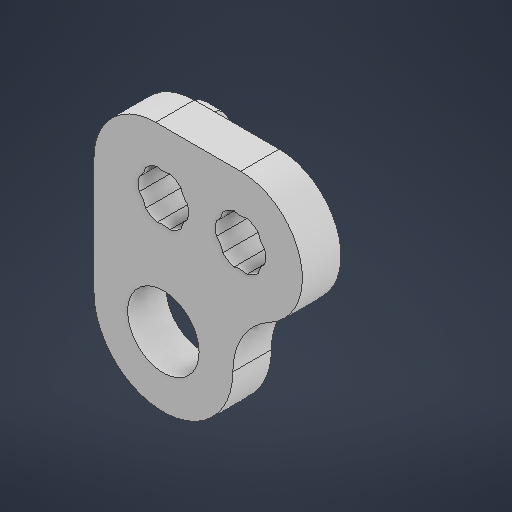
# Autodesk Inventor part: left_holder
Saved by Autodesk Inventor 2026.1 (Build 301233020, 233B)
## iProperties
Created: 2025-12-21
Part Number: left_holder
Material: Ogólny
Document SubType Name: Modeling
Designer: maciej
Density: 1 g/cm^3
Appearance: Domyślna
Author: maciej
Autodesk Inventor part; units mm, degrees
ref_plane "YZ Plane" through (0, 0, 0) normal (1, 0, 0) x (0, 1, 0)
ref_plane "XZ Plane" through (0, 0, 0) normal (0, 1, 0) x (-1, 0, 0)
ref_plane "XY Plane" through (0, 0, 0) normal (0, 0, 1) x (1, 0, 0)
sketch "Sketch1" plane through (0, 0, 0) normal (0, 0, 1) x (1, 0, 0)
  circle A0 centre (0, 0) radius 9.25
  circle A1 centre (0, 30) radius 6
  circle A2 centre (20, 30) radius 6
  circle A3 centre (0, 30) radius 6.5
  circle A4 centre (20, 30) radius 6.5
  arc A5 (-1.6614, 36.2841) -> (1.6614, 36.2841) centre (0, 41) ccw
  arc A6 (-6.2729, 31.7032) -> (-4.6115, 34.5808) centre (-9.5263, 35.5) ccw
  arc A7 (-4.6115, 25.4192) -> (-6.2729, 28.2968) centre (-9.5263, 24.5) ccw
  arc A8 (1.6614, 23.7159) -> (-1.6614, 23.7159) centre (0, 19) ccw
  arc A9 (6.2729, 28.2968) -> (4.6115, 25.4192) centre (9.5263, 24.5) ccw
  arc A10 (4.6115, 34.5808) -> (6.2729, 31.7032) centre (9.5263, 35.5) ccw
  arc A11 (18.3386, 36.2841) -> (21.6614, 36.2841) centre (20, 41) ccw
  arc A12 (13.7271, 31.7032) -> (15.3885, 34.5808) centre (10.4737, 35.5) ccw
  arc A13 (15.3885, 25.4192) -> (13.7271, 28.2968) centre (10.4737, 24.5) ccw
  arc A14 (21.6614, 23.7159) -> (18.3386, 23.7159) centre (20, 19) ccw
  arc A15 (26.2729, 28.2968) -> (24.6115, 25.4192) centre (29.5263, 24.5) ccw
  arc A16 (24.6115, 34.5808) -> (26.2729, 31.7032) centre (29.5263, 35.5) ccw
  circle A17 centre (0, 0) radius 18
  arc A18 (4.6562, 34.5353) -> (4.5, 33.9686) centre (20, 30) ccw
  arc A19 (27.5294, 15.8824) -> (20, 46) centre (20, 30) ccw
  line L0 (-18, 30) -> (-18, 0)
  line L1 (-2, 46) -> (20, 46)
  line L2 (-18, 0) -> (-13, 0)
  line L3 (-13, 0) -> (-13, 30)
  line L4 (-13, 30) -> (-18, 30)
  line L5 (-18, 30) -> (-18, 0)
  line L6 (-11.6913, 6.75) -> (0, 13.5)
  line L7 (0, 13.5) -> (11.6913, 6.75)
  line L8 (11.6913, 6.75) -> (11.6913, -6.75)
  line L9 (11.6913, -6.75) -> (0, -13.5)
  line L10 (0, -13.5) -> (-11.6913, -6.75)
  line L11 (-11.6913, -6.75) -> (-11.6913, 6.75)
  arc A20 (27.5294, 15.8824) -> (18, 0) centre (36, 0) ccw
  arc A21 (-2, 46) -> (-18, 30) centre (-2, 30) ccw
  point P0 (15.2791, 25.532)
  point P1 (15.5077, -9.1385)
  point P2 (-18, 30)
  point P3 (-1.6614, 23.7159)
  point P4 (1.6614, 23.7159)
  point P5 (-6.2729, 28.2968)
  point P6 (-4.6115, 25.4192)
  point P7 (-4.6115, 34.5808)
  point P8 (4.635, 34.4629)
  point P9 (6.2729, 31.7032)
  point P10 (18.3386, 23.7159)
  point P11 (21.6614, 23.7159)
  point P12 (13.7271, 31.7032)
  point P13 (26.2729, 31.7032)
  point P14 (15.3885, 25.4192)
  point P15 (15.3885, 34.5808)
  point P16 (4.6115, 25.4192)
  dimension "d1" = 12
  dimension "d0" = 18.5
  dimension "d2" = 30
  dimension "d3" = 12
  dimension "d4" = 20
  dimension "d5" = 13
  dimension "d6" = 13
  dimension "d7" = 5
  dimension "d10" = 360
  dimension "d12" = 5
  dimension "d15" = 360
  dimension "d17" = 36
  dimension "d21" = 16
  dimension "d25" = 5
  dimension "d26" = 30
  dimension "d32" = 27
  constraints: 41 point on circle, 24 end point, 21 centre point, 6 coincident, 6 tangent, 3 vertical alignment, 2 horizontal, 2 horizontal alignment, 2 parallel, 2 vertical, 1 equal radius, 1 perpendicular, 67 other
  measures "d0" diameter of A0
  measures "d2" distance of point (0, 0) point (0, 30)
  measures "d3" diameter of A2
  measures "d4" distance of A2.centre point (0, 30)
  measures "d5" diameter of A3
  measures "d6" diameter of A4
  measures "d7" radius of A5
  measures "d12" radius of A11
  measures "d17" diameter of A17
  measures "d21" radius of A19
  measures "d25" distance of L0.start L3.end
  measures "d26" distance of L3.end L2.end
  measures "d32" distance of L10.end L7.end
extrude "Extrusion1" add sketch "Sketch1" along normal blind 10 contours A10 A18 A3 | A9 A3 | A8 A3 | A5 A3 | A7 A3 | A6 A3 | A16 A4 | A15 A4 | A11 A4 | A14 A4 | A12 A4 | A13 A4 | L2 L3 A17 | L0 L4 L3 A17 | A17 L3 L2 | A17 L3 L4 A21 L1 A19 A20 | L6 L7 L8 L9 L10 L11 picked at (5.482, 33.1405)
extrude "Extrusion2" add sketch "Sketch1" against normal blind 20 contours L0 L4 L3 A17 | A17 L3 L2 picked at (-13.7089, 7.4021)
fillet "Fillet1" radius 5 2 edges at (-15.5, 30, -20) (-15.5, 0, -20)
sketch "Sketch2" plane through (-13, 0, 0) normal (1, 0, 0) x (0, 0, -1)
  line L0 (0, 30) -> (15, 30) projected
  line L1 (20, 25) -> (20, 5) projected
  line L2 (0, 0) -> (15, 0) projected
  point P0 (10, 20)
  point P1 (10, 10)
  dimension "d34" = 10
  dimension "d35" = 10
  dimension "d36" = 10
  dimension "d37" = 10
  measures "d34" distance from line of L0 point (10, 20)
  measures "d35" distance from line of L1 point (10, 20)
  measures "d36" distance from line of L2 point (10, 10)
  measures "d37" distance from line of L1 point (10, 10)
hole "Hole1" at (-13, 20, -10) at (-13, 10, -10) direction (-1, 0, 0) diameter 3 end through all
chamfer "Chamfer1" distance 5 distance2 15 2 edges at (-15.5, 30, 0) (-15.5, 0, 0) measured on face at (-15.5, -0.5, 0) measured on face at (-15.5, 30.5, 0)
chamfer "Chamfer2" distance 1 angle 45 1 edges at (-13, 15, 0)
body "Solid1"
